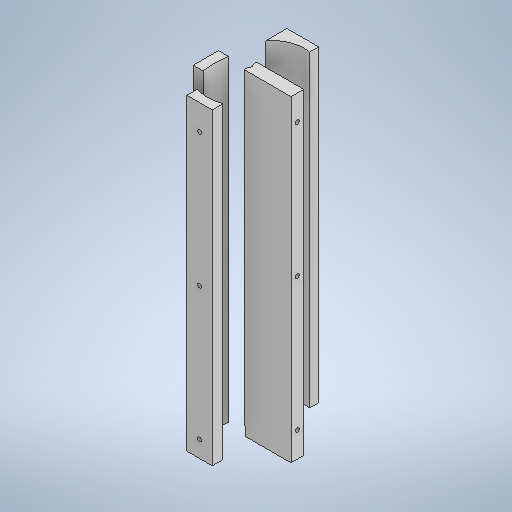
# Autodesk Inventor part: TS_V1_Fallmagazin_Wandung_int
Saved by Autodesk Inventor 2025.2 (Build 292293000, 293)
## iProperties
Created: 2025-06-10
Part Number: TS_V1_Fallmagazin_Wandung_int
Material: Generisch
Document SubType Name: Modeling
Designer: tino
Density: 1 g/cm^3
Appearance: Vorgabe
Author: tino
Autodesk Inventor part; units mm, degrees
ref_plane "YZ Plane" through (0, 0, 0) normal (1, 0, 0) x (0, 1, 0)
ref_plane "XZ Plane" through (0, 0, 0) normal (0, 1, 0) x (-1, 0, 0)
ref_plane "XY Plane" through (0, 0, 0) normal (0, 0, 1) x (1, 0, 0)
sketch "Skizze1" plane through (0, 0, 0) normal (0, 0, 1) x (1, 0, 0)
  spline S0 degree 3 poles (4.1682, 35.1897) (1.1905, 36.4598) (-2.2497, 35.1642) (-6.2549, 34.1582) (-11.7361, 32.1479) (-17.2675, 27.437) (-17.3979, 22.2805) (-19.1794, 11.8373) (-24.2043, -4.2198) (-21.9122, -21.3618) (-15.7263, -32.1361) (-8.9601, -34.8731) (-7.7344, -35.2068) knots 0 0 0 0 0.05535 0.076528 0.211782 0.295547 0.382964 0.432922 0.754884 0.81234 0.967238 1 1 1 1
  spline S1 degree 3 poles (-7.7344, -35.2068) (-2.4391, -36.6482) (4.9342, -35.145) (14.3889, -31.3641) (20.2206, -28.2766) (23.0847, -23.1792) (23.281, -18.9959) (17.3062, -16.4997) (13.7398, -19.2937) (6.9074, -22.9332) (-1.1986, -27.1621) (-10.3055, -22.9326) (-14.0352, -10.4002) (-9.4599, -0.926) (-6.8333, 0.3153) (-5.9182, 2.0588) (-5.9367, 4.1791) (-8.2887, 5.2306) (-8.3641, 10.4373) (-1.0106, 14.1251) (4.0821, 20.0507) (3.0635, 26.3026) (2.9493, 28.6136) (3.7888, 29.834) (5.5778, 31.0924) (6.6132, 32.7745) (5.2458, 34.7086) (4.2657, 35.1481) (4.1682, 35.1897) knots 0 0 0 0 0.14153 0.17035 0.245987 0.25892 0.290227 0.326265 0.372233 0.38898 0.482096 0.508256 0.624416 0.647418 0.715274 0.72607 0.746892 0.801722 0.811885 0.848514 0.916356 0.943374 0.948219 0.962959 0.96651 0.98188 0.998188 1 1 1 1
  arc A0 (-7.9107, 24.207) -> (-7.9109, 20.407) centre (-6.0635, 22.307) ccw
  line L0 (-7.9107, 24.207) -> (-4.2161, 24.2069)
  arc A1 (-4.2163, 20.4069) -> (-4.2161, 24.2069) centre (-6.0635, 22.307) ccw
  line L1 (-4.2163, 20.4069) -> (-7.9109, 20.407)
  spline S2 degree 3 poles (4.1682, 35.1897) (1.1905, 36.4598) (-2.2497, 35.1642) (-6.255, 34.1582) (-11.7361, 32.1479) (-17.2675, 27.437) (-17.3979, 22.2805) (-19.1794, 11.8373) (-24.2043, -4.2198) (-21.9122, -21.3619) (-15.7263, -32.1361) (-8.9601, -34.8731) (-7.7344, -35.2068) knots 0 0 0 0 0.05535 0.076528 0.211782 0.295547 0.382964 0.432922 0.754884 0.81234 0.967238 1 1 1 1
  spline S3 degree 3 poles (-7.7344, -35.2068) (-2.4391, -36.6482) (4.9342, -35.145) (14.3889, -31.3641) (20.2206, -28.2766) (23.0847, -23.1792) (23.281, -18.9959) (17.3062, -16.4997) (13.7398, -19.2937) (6.9074, -22.9332) (-1.1986, -27.1621) (-10.3055, -22.9326) (-14.0352, -10.4002) (-9.4599, -0.926) (-6.8333, 0.3153) (-5.9182, 2.0588) (-5.9367, 4.1791) (-8.2887, 5.2306) (-8.3641, 10.4373) (-1.0106, 14.1251) (4.0821, 20.0507) (3.0635, 26.3026) (2.9493, 28.6136) (3.7888, 29.834) (5.5778, 31.0924) (6.6132, 32.7745) (5.2458, 34.7086) (4.2657, 35.1481) (4.1682, 35.1897) knots 0 0 0 0 0.14153 0.17035 0.245987 0.25892 0.290227 0.326265 0.372233 0.38898 0.482096 0.508256 0.624416 0.647418 0.715274 0.72607 0.746892 0.801722 0.811885 0.848514 0.916356 0.943374 0.948219 0.962959 0.96651 0.98188 0.998188 1 1 1 1
  line L2 (-4.2163, 20.4069) -> (-7.9109, 20.407)
  arc A2 (-4.2163, 20.4069) -> (-4.2161, 24.2069) centre (-6.0635, 22.307) ccw
  line L3 (-7.9107, 24.207) -> (-4.2161, 24.2069)
  arc A3 (-7.9107, 24.207) -> (-7.9109, 20.407) centre (-6.0635, 22.307) ccw
  line L4 (-22.9949, 35.8296) -> (22.9949, 35.8296) construction
  line L5 (22.9949, 35.8296) -> (22.9949, -35.8296) construction
  line L6 (22.9949, -35.8296) -> (-22.9949, -35.8296) construction
  line L7 (-22.9949, -35.8296) -> (-22.9949, 35.8296) construction
  line L8 (-22.9949, 35.8296) -> (22.9949, -35.8296) construction
  line L9 (-22.9949, -35.8296) -> (22.9949, 35.8296) construction
  point P0 (0, 0)
  point P1 (-38.8867, -20.8658)
  point P2 (0, 0)
  constraints: 20 end point, 8 point on circle, 4 centre point, 3 horizontal, 3 perpendicular, 2 vertical, 1 midpoint, 8 other
sketch "Skizze2" plane through (0, 0, 0) normal (0, 0, 1) x (1, 0, 0)
  line L0 (-30, 42.5) -> (30, 42.5)
  line L1 (30, 42.5) -> (30, -42.5)
  line L2 (30, -42.5) -> (-30, -42.5)
  line L3 (-30, -42.5) -> (-30, 42.5)
  line L4 (-30, 42.5) -> (30, -42.5) construction
  line L5 (30, 42.5) -> (-30, -42.5) construction
  arc A0 (-7.9107, 24.207) -> (-7.9109, 20.407) centre (-6.0635, 22.307) ccw
  arc A1 (-7.9107, 24.207) -> (-7.9109, 20.407) centre (-6.0635, 22.307) ccw
  line L6 (-7.9107, 24.207) -> (-4.2161, 24.2069)
  line L7 (-7.9107, 24.207) -> (-4.2161, 24.2069)
  line L8 (-4.2163, 20.4069) -> (-7.9109, 20.407)
  line L9 (-4.2163, 20.4069) -> (-7.9109, 20.407)
  arc A2 (-4.2163, 20.4069) -> (-4.2161, 24.2069) centre (-6.0635, 22.307) ccw
  arc A3 (-4.2163, 20.4069) -> (-4.2161, 24.2069) centre (-6.0635, 22.307) ccw
  line L10 (-22.9949, 35.8296) -> (22.9949, 35.8296) construction
  line L11 (-22.9949, -35.8296) -> (-22.9949, 35.8296) construction
  spline S0 degree 3 poles (4.1682, 35.1897) (1.1905, 36.4598) (-2.2497, 35.1642) (-6.255, 34.1582) (-11.7361, 32.1479) (-17.2675, 27.437) (-17.3979, 22.2805) (-19.1794, 11.8373) (-24.2043, -4.2198) (-21.9122, -21.3619) (-15.7263, -32.1361) (-8.9601, -34.8731) (-7.7344, -35.2068) knots 0 0 0 0 0.05535 0.076528 0.211782 0.295547 0.382964 0.432922 0.754884 0.81234 0.967238 1 1 1 1
  spline S1 degree 3 poles (4.1682, 35.1897) (1.1905, 36.4598) (-2.2497, 35.1642) (-6.2549, 34.1582) (-11.7361, 32.1479) (-17.2675, 27.437) (-17.3979, 22.2805) (-19.1794, 11.8373) (-24.2043, -4.2198) (-21.9122, -21.3618) (-15.7263, -32.1361) (-8.9601, -34.8731) (-7.7344, -35.2068) knots 0 0 0 0 0.05535 0.076528 0.211782 0.295547 0.382964 0.432922 0.754884 0.81234 0.967238 1 1 1 1
  line L12 (-22.9949, 35.8296) -> (22.9949, -35.8296) construction
  line L13 (-22.9949, -35.8296) -> (22.9949, 35.8296) construction
  line L14 (22.9949, -35.8296) -> (-22.9949, -35.8296) construction
  spline S2 degree 3 poles (-7.7344, -35.2068) (-2.4391, -36.6482) (4.9342, -35.145) (14.3889, -31.3641) (20.2206, -28.2766) (23.0847, -23.1792) (23.281, -18.9959) (17.3062, -16.4997) (13.7398, -19.2937) (6.9074, -22.9332) (-1.1986, -27.1621) (-10.3055, -22.9326) (-14.0352, -10.4002) (-9.4599, -0.926) (-6.8333, 0.3153) (-5.9182, 2.0588) (-5.9367, 4.1791) (-8.2887, 5.2306) (-8.3641, 10.4373) (-1.0106, 14.1251) (4.0821, 20.0507) (3.0635, 26.3026) (2.9493, 28.6136) (3.7888, 29.834) (5.5778, 31.0924) (6.6132, 32.7745) (5.2458, 34.7086) (4.2657, 35.1481) (4.1682, 35.1897) knots 0 0 0 0 0.14153 0.17035 0.245987 0.25892 0.290227 0.326265 0.372233 0.38898 0.482096 0.508256 0.624416 0.647418 0.715274 0.72607 0.746892 0.801722 0.811885 0.848514 0.916356 0.943374 0.948219 0.962959 0.96651 0.98188 0.998188 1 1 1 1
  spline S3 degree 3 poles (-7.7344, -35.2068) (-2.4391, -36.6482) (4.9342, -35.145) (14.3889, -31.3641) (20.2206, -28.2766) (23.0847, -23.1792) (23.281, -18.9959) (17.3062, -16.4997) (13.7398, -19.2937) (6.9074, -22.9332) (-1.1986, -27.1621) (-10.3055, -22.9326) (-14.0352, -10.4002) (-9.4599, -0.926) (-6.8333, 0.3153) (-5.9182, 2.0588) (-5.9367, 4.1791) (-8.2887, 5.2306) (-8.3641, 10.4373) (-1.0106, 14.1251) (4.0821, 20.0507) (3.0635, 26.3026) (2.9493, 28.6136) (3.7888, 29.834) (5.5778, 31.0924) (6.6132, 32.7745) (5.2458, 34.7086) (4.2657, 35.1481) (4.1682, 35.1897) knots 0 0 0 0 0.14153 0.17035 0.245987 0.25892 0.290227 0.326265 0.372233 0.38898 0.482096 0.508256 0.624416 0.647418 0.715274 0.72607 0.746892 0.801722 0.811885 0.848514 0.916356 0.943374 0.948219 0.962959 0.96651 0.98188 0.998188 1 1 1 1
  line L15 (22.9949, 35.8296) -> (22.9949, -35.8296) construction
  line L16 (-40, 52.5) -> (40, 52.5)
  line L17 (40, 52.5) -> (40, -52.5)
  line L18 (40, -52.5) -> (-40, -52.5)
  line L19 (-40, -52.5) -> (-40, 52.5)
  line L20 (-40, 52.5) -> (40, -52.5) construction
  line L21 (40, 52.5) -> (-40, -52.5) construction
  point P0 (0, 0)
  point P1 (0, 0)
  point P2 (-38.8867, -20.8658)
  point P3 (0, 0)
  dimension "d0" = 45.9898
  dimension "d1" = 71.6591
  dimension "d2" = 60
  dimension "d3" = 85
  dimension "d4" = 80
  dimension "d5" = 105
  constraints: 24 end point, 4 midpoint, 4 parallel, 2 horizontal, 2 perpendicular
  measures "d0" distance between parallel lines of L15 L11
  measures "d1" distance of L11.start L10.start
  measures "d2" distance of L0.start L0.end
  measures "d3" distance of L2.end L0.start
  measures "d4" distance of L17.end L18.end
  measures "d5" distance of L16.end L17.end
sketch "Skizze5" plane through (0, 0, 0) normal (0, 0, 1) x (1, 0, 0)
  spline S0 degree 3 poles (4.1682, 35.1897) (1.1905, 36.4598) (-2.2497, 35.1642) (-6.255, 34.1582) (-11.7361, 32.1479) (-17.2675, 27.437) (-17.3979, 22.2805) (-19.1794, 11.8373) (-24.2043, -4.2198) (-21.9122, -21.3619) (-15.7263, -32.1361) (-8.9601, -34.8731) (-7.7344, -35.2068) knots 0 0 0 0 0.05535 0.076528 0.211782 0.295547 0.382964 0.432922 0.754884 0.81234 0.967238 1 1 1 1
  spline S1 degree 3 poles (-7.7344, -35.2068) (-2.4391, -36.6482) (4.9342, -35.145) (14.3889, -31.3641) (20.2206, -28.2766) (23.0847, -23.1792) (23.281, -18.9959) (17.3062, -16.4997) (13.7398, -19.2937) (6.9074, -22.9332) (-1.1986, -27.1621) (-10.3055, -22.9326) (-14.0352, -10.4002) (-9.4599, -0.926) (-6.8333, 0.3153) (-5.9182, 2.0588) (-5.9367, 4.1791) (-8.2887, 5.2306) (-8.3641, 10.4373) (-1.0106, 14.1251) (4.0821, 20.0507) (3.0635, 26.3026) (2.9493, 28.6136) (3.7888, 29.834) (5.5778, 31.0924) (6.6132, 32.7745) (5.2458, 34.7086) (4.2657, 35.1481) (4.1682, 35.1897) knots 0 0 0 0 0.14153 0.17035 0.245987 0.25892 0.290227 0.326265 0.372233 0.38898 0.482096 0.508256 0.624416 0.647418 0.715274 0.72607 0.746892 0.801722 0.811885 0.848514 0.916356 0.943374 0.948219 0.962959 0.96651 0.98188 0.998188 1 1 1 1
  line L0 (-4.2163, 20.4069) -> (-7.9109, 20.407)
  line L1 (-4.2163, 20.4069) -> (-7.9109, 20.407)
  arc A0 (-4.2163, 20.4069) -> (-4.2161, 24.2069) centre (-6.0635, 22.307) ccw
  arc A1 (-4.2163, 20.4069) -> (-4.2161, 24.2069) centre (-6.0635, 22.307) ccw
  line L2 (-7.9107, 24.207) -> (-4.2161, 24.2069)
  line L3 (-7.9107, 24.207) -> (-4.2161, 24.2069)
  arc A2 (-7.9107, 24.207) -> (-7.9109, 20.407) centre (-6.0635, 22.307) ccw
  arc A3 (-7.9107, 24.207) -> (-7.9109, 20.407) centre (-6.0635, 22.307) ccw
  arc A4 (-4.2163, 20.4069) -> (-4.2161, 24.2069) centre (-6.0635, 22.307) ccw
  arc A5 (-7.9107, 24.207) -> (-7.9109, 20.407) centre (-6.0635, 22.307) ccw
  arc A6 (-7.9107, 24.207) -> (-7.9109, 20.407) centre (-6.0635, 22.307) ccw
  line L4 (-4.2163, 20.4069) -> (-7.9109, 20.407)
  line L5 (-4.2163, 20.4069) -> (-7.9109, 20.407)
  line L6 (-7.9107, 24.207) -> (-4.2161, 24.2069)
  line L7 (-7.9107, 24.207) -> (-4.2161, 24.2069)
  arc A7 (-4.2163, 20.4069) -> (-4.2161, 24.2069) centre (-6.0635, 22.307) ccw
  spline S2 degree 3 poles (-7.7344, -35.2068) (-2.4391, -36.6482) (4.9342, -35.145) (14.3889, -31.3641) (20.2206, -28.2766) (23.0847, -23.1792) (23.281, -18.9959) (17.3062, -16.4997) (13.7398, -19.2937) (6.9074, -22.9332) (-1.1986, -27.1621) (-10.3055, -22.9326) (-14.0352, -10.4002) (-9.4599, -0.926) (-6.8333, 0.3153) (-5.9182, 2.0588) (-5.9367, 4.1791) (-8.2887, 5.2306) (-8.3641, 10.4373) (-1.0106, 14.1251) (4.0821, 20.0507) (3.0635, 26.3026) (2.9493, 28.6136) (3.7888, 29.834) (5.5778, 31.0924) (6.6132, 32.7745) (5.2458, 34.7086) (4.2657, 35.1481) (4.1682, 35.1897) knots 0 0 0 0 0.14153 0.17035 0.245987 0.25892 0.290227 0.326265 0.372233 0.38898 0.482096 0.508256 0.624416 0.647418 0.715274 0.72607 0.746892 0.801722 0.811885 0.848514 0.916356 0.943374 0.948219 0.962959 0.96651 0.98188 0.998188 1 1 1 1
  arc A8 (-22.1754, 0.5) -> (-22.1754, -19.5) centre (36.9854, -9.5) ccw
  line L8 (-22.1754, 0.5) -> (-30, 0.5)
  line L9 (-30, 0.5) -> (-30, -19.5)
  line L10 (-30, -19.5) -> (-22.1754, -19.5)
  line L11 (8, -34.1505) -> (8, -42.5)
  line L12 (8, -42.5) -> (-12, -42.5)
  line L13 (-12, -42.5) -> (-12, -34.1505)
  arc A9 (-12, -34.1505) -> (8, -34.1505) centre (-2, -5.8662) ccw
  line L14 (-7.0277, 4.9) -> (-7.0277, 7.6)
  line L15 (-7.0277, 7.6) -> (30, 7.6)
  line L16 (30, 7.6) -> (30, -2.4)
  line L17 (30, -2.4) -> (-7.0277, -2.4)
  line L18 (-7.0277, -2.4) -> (-7.0277, 0.3)
  arc A10 (-7.0277, 0.3) -> (-7.0277, 4.9) centre (-8.9539, 2.6) ccw
  line L19 (-30, -42.5) -> (-30, 42.5)
  line L20 (30, 42.5) -> (30, -42.5)
  line L21 (-30, 42.5) -> (30, 42.5)
  line L22 (30, -42.5) -> (-30, -42.5)
  line L23 (-18.1, 25.7505) -> (-18.1, 42.5)
  arc A11 (6.9, 35.3642) -> (-18.1, 25.7505) centre (1.977, 10.8537) ccw
  line L24 (-5.9589, 2.6) -> (30, 2.6) construction
  line L25 (6.9, 35.3642) -> (6.9, 42.5)
  point P0 (0, 0)
  point P1 (-30, -9.5)
  point P2 (-5.6, 42.5)
  point P3 (-2, -42.5)
  dimension "d31" = 20
  dimension "d34" = 60
  dimension "d38" = 20
  dimension "d39" = 30
  dimension "d43" = 2.7
  dimension "d45" = 10
  dimension "d46" = 3
  dimension "d49" = 25
  dimension "d57" = 5
  dimension "d120" = 33
  dimension "d121" = 28
  dimension "d124" = 24.4
  dimension "d125" = 39.9
  dimension "d126" = 8.3495
  dimension "d129" = 25
  dimension "d130" = 12.5
  constraints: 29 end point, 12 perpendicular, 8 point on circle, 5 point on line, 4 centre point, 3 collinear, 3 equal length, 2 horizontal, 2 midpoint, 1 parallel, 1 vertical, 6 other
  measures "d31" distance of L8.end L9.end
  measures "d34" radius of A8
  measures "d38" distance of L11.end L12.end
  measures "d39" radius of A9
  measures "d43" distance of L14.start L14.end
  measures "d45" distance between parallel lines of L17 L15
  measures "d46" radius of A10
  measures "d49" radius of A11
  measures "d57" distance between parallel lines of L24 L15
  measures "d120" distance from line of point (-30, -9.5) L22
  measures "d121" distance from line of point (-2, -42.5) L19
  measures "d124" distance from line of L19 point (-5.6, 42.5)
  measures "d125" distance from line of L21 L24.end
  measures "d126" distance of L11.start L11.end
  measures "d129" distance between parallel lines of L25 L23
  measures "d130" distance from line of L23 point (-5.6, 42.5)
extrude "Extrusion3" add sketch "Skizze5" along normal blind 250 contours A11 L23 L21 L25 | A10 L14 L15 L16 L17 L18 | A9 L11 L12 L13 | A8 L10 L9 L8
sketch "Skizze6" plane through (30, -2.4, 0) normal (1, 0, 0) x (0, 0, -1)
  line L0 (0, 0) -> (-250, 0) projected
  line L1 (0, 10) -> (-250, 10) projected
  line L2 (0, 54.9) -> (0, -50.1) projected
  line L3 (-250, 0) -> (-250, 10) projected
  point P0 (0, 2.4)
  point P1 (-230, 5)
  point P2 (-125, 5)
  point P3 (-20, 5)
  dimension "d61" = 10
  dimension "d62" = 5
  dimension "d64" = 20
  dimension "d131" = 20
  constraints: 2 horizontal alignment
  measures "d61" distance of L0.end L1.end
  measures "d62" distance from line of point (-230, 5) L1
  measures "d64" distance from line of L2 point (-20, 5)
  measures "d131" horizontal distance of point (-230, 5) L1.end
sketch "Skizze7" plane through (-12, -42.5, 0) normal (0, -1, 0) x (1, 0, 0)
  line L0 (0, 0) -> (0, 250) projected
  line L1 (20, 0) -> (20, 250) projected
  line L2 (0, 250) -> (20, 250) projected
  line L3 (0, 0) -> (20, 0) projected
  point P0 (12, 0)
  point P1 (10, 230)
  point P2 (10, 125)
  point P3 (10, 20)
  dimension "d65" = 20
  dimension "d66" = 10
  dimension "d67" = 20
  dimension "d68" = 20
  dimension "d74" = 125
  constraints: 2 vertical alignment
  measures "d65" distance between parallel lines of L0 L1
  measures "d66" distance from line of L0 point (10, 230)
  measures "d67" distance from line of L2 point (10, 230)
  measures "d68" distance from line of L3 point (10, 20)
  measures "d74" distance from line of L2 point (10, 125)
sketch "Skizze8" plane through (-30, -19.5, 0) normal (-1, 0, 0) x (0, 0, 1)
  line L0 (0, 20) -> (0, 0) projected
  line L1 (0, 0) -> (250, 0) projected
  line L2 (250, 20) -> (250, 0) projected
  line L3 (0, 20) -> (250, 20) projected
  point P0 (0, 19.5)
  point P1 (230, 10)
  point P2 (125, 10)
  point P3 (20, 10)
  point P4 (250, 10)
  dimension "d69" = 20
  dimension "d70" = 10
  dimension "d71" = 20
  dimension "d72" = 20
  dimension "d73" = 125
  constraints: 2 horizontal alignment, 1 midpoint
  measures "d69" distance of L2.start L1.end
  measures "d70" distance from line of point (230, 10) L3
  measures "d71" distance from line of L2 point (230, 10)
  measures "d72" distance from line of L0 point (20, 10)
  measures "d73" distance of point (125, 10) point (250, 10)
sketch "Skizze9" plane through (-18.1, 42.5, 0) normal (0, 1, 0) x (1, 0, 0)
  line L0 (25, 0) -> (0, 0) projected
  line L1 (25, -250) -> (0, -250) projected
  line L2 (0, 0) -> (0, -250) projected
  line L3 (25, 0) -> (25, -250) projected
  point P0 (18.1, 0)
  point P1 (12.5, -230)
  point P2 (12.5, -125)
  point P3 (12.5, -20)
  dimension "d78" = 20
  dimension "d79" = 20
  dimension "d80" = 125
  constraints: 2 vertical alignment
  measures "d78" distance from line of point (12.5, -230) L1
  measures "d79" distance from line of L0 point (12.5, -20)
  measures "d80" distance from line of point (12.5, -125) L1
hole "Bohrung2" at (-5.6, 42.5, 230) at (-5.6, 42.5, 125) at (-5.6, 42.5, 20) direction (0, -1, 0) diameter 3.242 depth 6 tip angle 118 thread size "M4x0.7" class "6H" standard "ISO Metric profile"
hole "Bohrung4" at (-30, -9.5, 230) at (-30, -9.5, 125) at (-30, -9.5, 20) direction (1, 0, 0) diameter 3.242 depth 6 tip angle 118 thread size "M4x0.7" class "6H" standard "ISO Metric profile"
hole "Bohrung5" at (-2, -42.5, 230) at (-2, -42.5, 125) at (-2, -42.5, 20) direction (0, 1, 0) diameter 3.242 depth 6 tip angle 118 thread size "M4x0.7" class "6H" standard "ISO Metric profile"
hole "Bohrung6" at (30, 2.6, 230) at (30, 2.6, 125) at (30, 2.6, 20) direction (-1, 0, 0) diameter 3.242 depth 11 tip angle 118 thread size "M4x0.7" class "6H" standard "ISO Metric profile"
sketch "Skizze10" plane through (0, 0, 0) normal (0, 0, -1) x (-1, 0, 0)
  arc A0 (7.0277, 4.9) -> (7.0277, 0.3) centre (8.9539, 2.6) ccw projected
  arc A1 (7.0277, 4.9) -> (7.0277, 0.3) centre (8.9539, 2.6) ccw projected
  line L0 (7.0277, 0.3) -> (7.0277, -2.4) projected
  line L1 (7.0277, 0.3) -> (7.0277, -2.4) projected
  line L2 (7.0277, -2.4) -> (-30, -2.4) projected
  line L3 (7.0277, -2.4) -> (-30, -2.4) projected
  line L4 (-30, -2.4) -> (-30, 7.6) projected
  line L5 (7.0277, 7.6) -> (7.0277, 4.9) projected
  line L6 (7.0277, 7.6) -> (7.0277, 4.9) projected
  line L7 (-30, 7.6) -> (7.0277, 7.6) projected
  line L8 (-30, 7.6) -> (7.0277, 7.6) projected
  line L9 (-30, 7.6) -> (7.0277, 7.6) projected
  line L10 (-30, 7.6) -> (7.0277, 7.6) projected
  line L11 (7.0277, -2.4) -> (-30, -2.4) projected
  line L12 (7.0277, -2.4) -> (-30, -2.4) projected
  arc A2 (7.0277, 4.9) -> (7.0277, 0.3) centre (8.9539, 2.6) ccw projected
  line L13 (7.0277, 0.3) -> (7.0277, -2.4) projected
  line L14 (7.0277, -2.4) -> (-30, -2.4) projected
  line L15 (-30, -2.4) -> (-30, 7.6) projected
  line L16 (-30, 7.6) -> (7.0277, 7.6) projected
  line L17 (7.0277, 7.6) -> (7.0277, 4.9) projected
  line L18 (-19, 4.221) -> (-19, 0.979) projected
  line L19 (-19, 4.221) -> (-19, 0.979) projected
  line L20 (-19, 4.221) -> (-19, 0.979) projected
  line L21 (-19, 4.221) -> (-19, 0.979) projected
  line L22 (-19, 4.221) -> (-19, 0.979) projected
  line L23 (-30, 0.979) -> (-30, 4.221) projected
  line L24 (-30, 0.979) -> (-30, 4.221) projected
  line L25 (-30, -2.4) -> (-30, 7.6) projected
  line L26 (-30, 0.979) -> (-30, 4.221) projected
  line L27 (-30, 0.979) -> (-30, 4.221) projected
  line L28 (-30, 0.979) -> (-30, 4.221) projected
  line L29 (-30, -2.4) -> (-30, 7.6) projected
  line L30 (-30, -2.4) -> (-30, 7.6) projected
  line L31 (-6.9, 35.3642) -> (-6.9, 42.5) projected
  line L32 (-6.9, 35.3642) -> (-6.9, 42.5) projected
  line L33 (-6.9, 35.3642) -> (-6.9, 42.5) projected
  line L34 (7.221, 36.5) -> (3.979, 36.5) projected
  line L35 (3.979, 42.5) -> (7.221, 42.5) projected
  arc A3 (18.1, 25.7505) -> (-6.9, 35.3642) centre (-1.977, 10.8537) ccw projected
  arc A4 (18.1, 25.7505) -> (-6.9, 35.3642) centre (-1.977, 10.8537) ccw projected
  arc A5 (18.1, 25.7505) -> (-6.9, 35.3642) centre (-1.977, 10.8537) ccw projected
  line L36 (3.979, 42.5) -> (7.221, 42.5) projected
  line L37 (3.979, 42.5) -> (7.221, 42.5) projected
  line L38 (3.979, 42.5) -> (7.221, 42.5) projected
  line L39 (-6.9, 42.5) -> (18.1, 42.5) projected
  line L40 (-6.9, 42.5) -> (18.1, 42.5) projected
  line L41 (-30, 42.5) -> (18.1, 42.5) projected
  line L42 (18.1, 42.5) -> (18.1, 25.7505) projected
  line L43 (18.1, 42.5) -> (18.1, 25.7505) projected
  line L44 (18.1, 42.5) -> (18.1, 25.7505) projected
  line L45 (-19, 4.221) -> (-19, 0.979) projected
  line L46 (-30, 0.979) -> (-30, 4.221) projected
  line L47 (-19, 4.221) -> (-19, 0.979) projected
  line L48 (7.221, 36.5) -> (3.979, 36.5) projected
  line L49 (-6.9, 35.3642) -> (-6.9, 42.5) projected
  arc A6 (18.1, 25.7505) -> (-6.9, 35.3642) centre (-1.977, 10.8537) ccw projected
  line L50 (-30, 42.5) -> (18.1, 42.5) projected
  line L51 (18.1, 42.5) -> (18.1, 25.7505) projected
  line L52 (3.979, 42.5) -> (7.221, 42.5) projected
  arc A7 (22.1754, -19.5) -> (22.1754, 0.5) centre (-36.9854, -9.5) ccw projected
  arc A8 (22.1754, -19.5) -> (22.1754, 0.5) centre (-36.9854, -9.5) ccw projected
  line L53 (22.1754, 0.5) -> (30, 0.5) projected
  line L54 (22.1754, 0.5) -> (30, 0.5) projected
  line L55 (30, 0.5) -> (30, -19.5) projected
  line L56 (30, 0.5) -> (30, -19.5) projected
  line L57 (30, -19.5) -> (22.1754, -19.5) projected
  line L58 (30, -19.5) -> (22.1754, -19.5) projected
  line L59 (30, -7.879) -> (30, -11.121) projected
  line L60 (24, -11.121) -> (24, -7.879) projected
  line L61 (30, -7.879) -> (30, -11.121) projected
  line L62 (24, -11.121) -> (24, -7.879) projected
  line L63 (30, -7.879) -> (30, -11.121) projected
  line L64 (24, -11.121) -> (24, -7.879) projected
  line L65 (7.0277, 7.6) -> (7.0277, 4.9) projected
  line L66 (7.0277, 7.6) -> (7.0277, 4.9) projected
  arc A9 (7.0277, 4.9) -> (7.0277, 0.3) centre (8.9539, 2.6) ccw projected
  arc A10 (7.0277, 4.9) -> (7.0277, 0.3) centre (8.9539, 2.6) ccw projected
  line L67 (22.1754, 0.5) -> (30, 0.5) projected
  line L68 (22.1754, 0.5) -> (30, 0.5) projected
  line L69 (24, -11.121) -> (24, -7.879) projected
  arc A11 (22.1754, -19.5) -> (22.1754, 0.5) centre (-36.9854, -9.5) ccw projected
  arc A12 (22.1754, -19.5) -> (22.1754, 0.5) centre (-36.9854, -9.5) ccw projected
  line L70 (30, -7.879) -> (30, -11.121) projected
  line L71 (30, -7.879) -> (30, -11.121) projected
  line L72 (30, -7.879) -> (30, -11.121) projected
  line L73 (30, 0.5) -> (30, -19.5) projected
  line L74 (30, 0.5) -> (30, -19.5) projected
  line L75 (30, -19.5) -> (22.1754, -19.5) projected
  line L76 (30, -19.5) -> (22.1754, -19.5) projected
  line L77 (7.0277, 0.3) -> (7.0277, -2.4) projected
  line L78 (7.0277, 0.3) -> (7.0277, -2.4) projected
  line L79 (12, -34.1505) -> (12, -42.5) projected
  line L80 (12, -34.1505) -> (12, -42.5) projected
  line L81 (12, -42.5) -> (-8, -42.5) projected
  line L82 (12, -42.5) -> (-8, -42.5) projected
  line L83 (-8, -42.5) -> (-8, -34.1505) projected
  line L84 (-8, -42.5) -> (-8, -34.1505) projected
  arc A13 (-8, -34.1505) -> (12, -34.1505) centre (2, -5.8662) ccw projected
  arc A14 (-8, -34.1505) -> (12, -34.1505) centre (2, -5.8662) ccw projected
  line L85 (3.621, -42.5) -> (0.379, -42.5) projected
  line L86 (0.379, -36.5) -> (3.621, -36.5) projected
  line L87 (3.621, -42.5) -> (0.379, -42.5) projected
  line L88 (0.379, -36.5) -> (3.621, -36.5) projected
  line L89 (3.621, -42.5) -> (0.379, -42.5) projected
  line L90 (0.379, -36.5) -> (3.621, -36.5) projected
  arc A15 (-8, -34.1505) -> (12, -34.1505) centre (2, -5.8662) ccw projected
  arc A16 (-8, -34.1505) -> (12, -34.1505) centre (2, -5.8662) ccw projected
  line L91 (0.379, -36.5) -> (3.621, -36.5) projected
  line L92 (12, -34.1505) -> (12, -42.5) projected
  line L93 (12, -34.1505) -> (12, -42.5) projected
  line L94 (12, -34.1505) -> (12, -42.5) projected
  line L95 (12, -42.5) -> (-8, -42.5) projected
  line L96 (-8, -42.5) -> (-8, -34.1505) projected
  arc A17 (-8, -34.1505) -> (12, -34.1505) centre (2, -5.8662) ccw projected
  line L97 (3.621, -42.5) -> (0.379, -42.5) projected
  line L98 (3.621, -42.5) -> (0.379, -42.5) projected
  line L99 (3.621, -42.5) -> (0.379, -42.5) projected
  line L100 (12, -42.5) -> (-8, -42.5) projected
  line L101 (12, -42.5) -> (-8, -42.5) projected
  line L102 (-8, -42.5) -> (-8, -34.1505) projected
  line L103 (-8, -42.5) -> (-8, -34.1505) projected
  line L104 (3.621, -42.5) -> (0.379, -42.5) projected
  line L105 (0.379, -36.5) -> (3.621, -36.5) projected
  line L106 (3.979, 42.5) -> (7.221, 42.5) projected
  line L107 (0.379, -36.5) -> (3.621, -36.5) projected
  line L108 (30, -7.879) -> (30, -11.121) projected
  line L109 (24, -11.121) -> (24, -7.879) projected
  line L110 (0.379, -36.5) -> (3.621, -36.5) projected
  line L111 (3.621, -42.5) -> (0.379, -42.5) projected
  line L112 (0.379, -36.5) -> (3.621, -36.5) projected
  line L113 (12, -34.1505) -> (12, -42.5) projected
  arc A18 (-8, -34.1505) -> (12, -34.1505) centre (2, -5.8662) ccw projected
  line L114 (-8, -42.5) -> (-8, -34.1505) projected
  line L115 (12, -42.5) -> (-8, -42.5) projected
  arc A19 (22.1754, -19.5) -> (22.1754, 0.5) centre (-36.9854, -9.5) ccw projected
  line L116 (30, -19.5) -> (22.1754, -19.5) projected
  line L117 (30, 0.5) -> (30, -19.5) projected
  line L118 (22.1754, 0.5) -> (30, 0.5) projected
  line L119 (7.221, 36.5) -> (3.979, 36.5) projected
  line L120 (-6.9, 42.5) -> (18.1, 42.5) projected
  arc A20 (22.1754, -19.5) -> (22.1754, 0.5) centre (-36.9854, -9.5) ccw projected
  line L121 (22.1754, 0.5) -> (30, 0.5) projected
  line L122 (30, 0.5) -> (30, -19.5) projected
  line L123 (30, -19.5) -> (22.1754, -19.5) projected
  line L124 (7.221, 36.5) -> (3.979, 36.5) projected
  line L125 (3.979, 42.5) -> (7.221, 42.5) projected
  line L126 (7.221, 36.5) -> (3.979, 36.5) projected
  line L127 (30, -7.879) -> (30, -11.121) projected
  line L128 (24, -11.121) -> (24, -7.879) projected
  line L129 (30, -7.879) -> (30, -11.121) projected
  line L130 (24, -11.121) -> (24, -7.879) projected
  line L131 (24, -11.121) -> (24, -7.879) projected
  line L132 (3.979, 42.5) -> (7.221, 42.5) projected
  line L133 (7.221, 36.5) -> (3.979, 36.5) projected
  line L134 (7.221, 36.5) -> (3.979, 36.5) projected
  line L135 (-19, 4.221) -> (-19, 0.979) projected
  arc A21 (7.0277, 4.9) -> (7.0277, 0.3) centre (8.9539, 2.6) ccw projected
  line L136 (7.0277, 7.6) -> (7.0277, 4.9) projected
  line L137 (-30, 7.6) -> (7.0277, 7.6) projected
  line L138 (-30, -2.4) -> (-30, 7.6) projected
  line L139 (7.0277, -2.4) -> (-30, -2.4) projected
  line L140 (7.0277, 0.3) -> (7.0277, -2.4) projected
  line L141 (-6.9, 42.5) -> (18.1, 42.5) projected
  line L142 (3.979, 42.5) -> (7.221, 42.5) projected
  line L143 (7.221, 36.5) -> (3.979, 36.5) projected
  line L144 (-19, 4.221) -> (-19, 0.979) projected
  line L145 (24, -11.121) -> (24, -7.879) projected
  line L146 (3.621, -42.5) -> (0.379, -42.5) projected
  line L147 (0.379, -36.5) -> (3.621, -36.5) projected
  line L148 (7.221, 36.5) -> (3.979, 36.5) projected
  line L149 (23.0146, -19.5) -> (23.0146, -9.5)
  line L150 (5.9539, -2.4) -> (5.9539, 2.6)
  line L151 (-6.9, 35.3642) -> (-6.9, 42.5) projected
  arc A22 (18.1, 25.7505) -> (-6.9, 35.3642) centre (-1.977, 10.8537) ccw projected
  line L152 (18.1, 42.5) -> (18.1, 25.7505) projected
  line L153 (18.1, 42.5) -> (18.1, 25.7505) projected
  arc A23 (18.1, 25.7505) -> (-6.9, 35.3642) centre (-1.977, 10.8537) ccw projected
  line L154 (-6.9, 35.3642) -> (-6.9, 42.5) projected
  line L155 (0.379, -36.5) -> (3.621, -36.5) projected
  line L156 (0.379, -36.5) -> (3.621, -36.5) projected
  line L157 (0.379, -36.5) -> (3.621, -36.5) projected
  point P0 (0, 0)
  point P1 (-18.026, 2.6)
  point P2 (-18.026, 2.6)
  point P3 (23.026, -9.5)
  point P4 (5.6, 35.526)
  point P5 (23.026, -9.5)
  point P6 (5.6, 35.526)
  point P7 (-18.026, 2.6)
  point P8 (23.026, -9.5)
  point P9 (5.6, 35.526)
  point P10 (5.9539, 2.6)
  point P11 (23.0146, -19.5)
  point P12 (23.0146, -9.5)
  point P13 (2.5576, -35.8611)
  point P14 (2.5576, -35.8611)
  point P15 (2.5576, -35.8611)
  constraints: 4 end point, 2 point on circle, 2 point on line, 2 tangent, 2 vertical, 8 other
extrude "Extrusion4" cut sketch "Skizze10" against normal blind 7 contours A0 L0 L2 L150 | A7 L149 L57
sketch "Skizze11" plane through (0, 0, 0) normal (0, 0, -1) x (-1, 0, 0)
  line L0 (0.379, -36.5) -> (3.621, -36.5) projected
  line L1 (12, -34.1505) -> (12, -42.5) projected
  line L2 (12, -34.1505) -> (12, -42.5) projected
  line L3 (0.379, -36.5) -> (3.621, -36.5) projected
  line L4 (0.379, -36.5) -> (3.621, -36.5) projected
  line L5 (3.621, -42.5) -> (0.379, -42.5) projected
  line L6 (3.621, -42.5) -> (0.379, -42.5) projected
  line L7 (3.621, -42.5) -> (0.379, -42.5) projected
  line L8 (3.621, -42.5) -> (0.379, -42.5) projected
  line L9 (12, -42.5) -> (-8, -42.5) projected
  line L10 (12, -42.5) -> (-8, -42.5) projected
  line L11 (-8, -42.5) -> (-8, -34.1505) projected
  line L12 (-8, -42.5) -> (-8, -34.1505) projected
  arc A0 (-8, -34.1505) -> (12, -34.1505) centre (2, -5.8662) ccw projected
  arc A1 (-8, -34.1505) -> (12, -34.1505) centre (2, -5.8662) ccw projected
  line L13 (3.621, -42.5) -> (0.379, -42.5) projected
  line L14 (0.379, -36.5) -> (3.621, -36.5) projected
  line L15 (0.379, -36.5) -> (3.621, -36.5) projected
  line L16 (3.621, -42.5) -> (0.379, -42.5) projected
  line L17 (0.379, -36.5) -> (3.621, -36.5) projected
  line L18 (3.621, -42.5) -> (0.379, -42.5) projected
  line L19 (0.379, -36.5) -> (3.621, -36.5) projected
  line L20 (-8, -42.5) -> (-8, -34.1505) projected
  line L21 (12, -42.5) -> (-8, -42.5) projected
  arc A2 (-8, -34.1505) -> (12, -34.1505) centre (2, -5.8662) ccw projected
  line L22 (12, -34.1505) -> (12, -42.5) projected
  line L23 (12, -42.5) -> (-8, -42.5) projected
  line L24 (-8, -42.5) -> (-8, -34.1505) projected
  arc A3 (-8, -34.1505) -> (12, -34.1505) centre (2, -5.8662) ccw projected
  line L25 (12, -34.1505) -> (12, -42.5) projected
  line L26 (3.621, -42.5) -> (0.379, -42.5) projected
  line L27 (0.379, -36.5) -> (3.621, -36.5) projected
  line L28 (3.621, -42.5) -> (0.379, -42.5) projected
  line L29 (0.379, -36.5) -> (3.621, -36.5) projected
  line L30 (12, -34.1505) -> (12, -42.5) projected
  line L31 (12, -42.5) -> (-8, -42.5) projected
  line L32 (12, -34.1505) -> (12, -42.5) projected
  arc A4 (-8, -34.1505) -> (12, -34.1505) centre (2, -5.8662) ccw projected
  line L33 (-8, -42.5) -> (-8, -34.1505) projected
  line L34 (12, -42.5) -> (-8, -42.5) projected
  line L35 (-8, -42.5) -> (-8, -34.1505) projected
  arc A5 (-8, -34.1505) -> (12, -34.1505) centre (2, -5.8662) ccw projected
  line L36 (-6.9, 35.3642) -> (-6.9, 42.5) projected
  line L37 (-6.9, 35.3642) -> (-6.9, 42.5) projected
  line L38 (-30, 42.5) -> (30, 42.5) projected
  line L39 (-30, 42.5) -> (30, 42.5) projected
  line L40 (18.1, 42.5) -> (18.1, 25.7505) projected
  line L41 (18.1, 42.5) -> (18.1, 25.7505) projected
  arc A6 (18.1, 25.7505) -> (-6.9, 35.3642) centre (-1.977, 10.8537) ccw projected
  arc A7 (18.1, 25.7505) -> (-6.9, 35.3642) centre (-1.977, 10.8537) ccw projected
  line L42 (3.979, 42.5) -> (7.221, 42.5) projected
  line L43 (7.221, 36.5) -> (3.979, 36.5) projected
  line L44 (3.979, 42.5) -> (7.221, 42.5) projected
  line L45 (7.221, 36.5) -> (3.979, 36.5) projected
  line L46 (3.979, 42.5) -> (7.221, 42.5) projected
  line L47 (7.221, 36.5) -> (3.979, 36.5) projected
  arc A8 (18.1, 25.7505) -> (-6.9, 35.3642) centre (-1.977, 10.8537) ccw projected
  arc A9 (18.1, 25.7505) -> (-6.9, 35.3642) centre (-1.977, 10.8537) ccw projected
  line L48 (-6.9, 42.5) -> (18.1, 42.5) projected
  line L49 (18.1, 42.5) -> (18.1, 25.7505) projected
  line L50 (18.1, 42.5) -> (18.1, 25.7505) projected
  line L51 (-6.9, 35.3642) -> (-6.9, 42.5) projected
  line L52 (-6.9, 35.3642) -> (-6.9, 42.5) projected
  line L53 (3.979, 42.5) -> (7.221, 42.5) projected
  line L54 (3.979, 42.5) -> (7.221, 42.5) projected
  line L55 (3.979, 42.5) -> (7.221, 42.5) projected
  line L56 (-6.9, 42.5) -> (18.1, 42.5) projected
  line L57 (-6.9, 42.5) -> (18.1, 42.5) projected
  line L58 (3.979, 42.5) -> (7.221, 42.5) projected
  line L59 (7.221, 36.5) -> (3.979, 36.5) projected
  line L60 (7.221, 36.5) -> (3.979, 36.5) projected
  line L61 (3.979, 42.5) -> (7.221, 42.5) projected
  line L62 (7.221, 36.5) -> (3.979, 36.5) projected
  line L63 (7.221, 36.5) -> (3.979, 36.5) projected
  line L64 (-6.9, 42.5) -> (18.1, 42.5) projected
  line L65 (3.979, 42.5) -> (7.221, 42.5) projected
  line L66 (7.221, 36.5) -> (3.979, 36.5) projected
  line L67 (7.221, 36.5) -> (3.979, 36.5) projected
  line L68 (18.1, 42.5) -> (18.1, 25.7505) projected
  arc A10 (18.1, 25.7505) -> (-6.9, 35.3642) centre (-1.977, 10.8537) ccw projected
  line L69 (-6.9, 35.3642) -> (-6.9, 42.5) projected
  line L70 (-6.9, 35.3642) -> (-6.9, 42.5) projected
  arc A11 (18.1, 25.7505) -> (-6.9, 35.3642) centre (-1.977, 10.8537) ccw projected
  line L71 (18.1, 42.5) -> (18.1, 25.7505) projected
  line L72 (0.379, -36.5) -> (3.621, -36.5) projected
  line L73 (0.379, -36.5) -> (3.621, -36.5) projected
  line L74 (0.379, -36.5) -> (3.621, -36.5) projected
  point P0 (0, 0)
  point P1 (5.6, 35.526)
  point P2 (5.6, 35.526)
  point P3 (5.6, 35.526)
  point P4 (12, -34.1505)
  point P5 (-8, -34.1505)
  point P6 (2.5576, -35.8611)
  point P7 (2.5576, -35.8611)
  point P8 (2.5576, -35.8611)
  constraints: 10 other
extrude "Extrusion5" cut sketch "Skizze11" against normal blind 7
equation "\"d2\" = Breite_innen"
equation "\"d3\" = Laenge_innen"
equation "\"d4\" = Breite_aussen"
equation "\"d5\" = Laenge_aussen"
equation "\"d57\" = 0.5 * d45"
equation "\"d59\" = Hoehe_Magazin"
equation "\"d62\" = 0.5 * d61"
equation "\"d64\" = Abstand_Rand"
equation "\"d66\" = 0.5 * d65"
equation "\"d67\" = Abstand_Rand"
equation "\"d68\" = d67"
equation "\"d74\" = 0.5 * Hoehe_Magazin"
equation "\"d70\" = 0.5 * d69"
equation "\"d71\" = Abstand_Rand"
equation "\"d72\" = d71"
equation "\"d73\" = 0.5 * Hoehe_Magazin"
equation "\"d78\" = Abstand_Rand"
equation "\"d79\" = d78"
equation "\"d80\" = 0.5 * Hoehe_Magazin"
equation "\"d82\" = Bohrungstiefe_duenn"
equation "\"d96\" = Bohrungstiefe_duenn"
equation "\"d103\" = Bohrungstiefe_duenn"
equation "\"d110\" = Bohrungstiefe_tief"
equation "\"d116\" = Ausschubhoehe"
equation "\"d118\" = Ausschubhoehe"
equation "\"Breite_innen\" = 60"
equation "\"Laenge_innen\" = 85"
equation "\"Breite_aussen\" = Breite_innen + 2 * Wanddicke"
equation "\"Laenge_aussen\" = Laenge_innen + 2 * Wanddicke"
equation "\"Hoehe_Magazin\" = 250"
equation "\"Ausschubhoehe\" = 7"
equation "\"Absatz\" = 2"
equation "\"Abstand_Rand\" = 20"
equation "\"Bohrungstiefe_duenn\" = 5"
equation "\"Bohrungstiefe_tief\" = 10"
equation "\"Wanddicke\" = 10"
